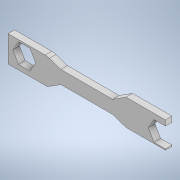
# Autodesk Inventor part: Whack01
Saved by Autodesk Inventor 2020.2 (Build 242310000, 310)
## iProperties
Created: 2019-11-16
Part Number: Whack01
Material: Generic
Document SubType Name: Modeling
Designer: steele
Density: 1 g/cm^3
Appearance: Default
Author: steele
Autodesk Inventor part; units mm, degrees
ref_plane "YZ Plane" through (0, 0, 0) normal (1, 0, 0) x (0, 1, 0)
ref_plane "XZ Plane" through (0, 0, 0) normal (0, 1, 0) x (-1, 0, 0)
ref_plane "XY Plane" through (0, 0, 0) normal (0, 0, 1) x (1, 0, 0)
sketch "Sketch1" plane through (0, 0, 0) normal (0, 0, 1) x (1, 0, 0)
  line L0 (76.176, -10.7873) -> (76.176, 14.6127)
  line L1 (-76.176, 10.7873) -> (-76.176, -14.6127)
  line L2 (-76.176, -14.6127) -> (76.176, 14.6127) construction
  line L3 (76.176, -10.7873) -> (-76.176, 10.7873) construction
  line L4 (76.176, 9.4269) -> (81.6753, -0.0981)
  line L5 (81.6753, -0.0981) -> (76.176, -9.6231)
  line L6 (76.176, -9.6231) -> (65.1775, -9.6231)
  line L7 (65.1775, -9.6231) -> (59.6782, -0.0981)
  line L8 (59.6782, -0.0981) -> (65.1775, 9.4269)
  line L9 (65.1775, 9.4269) -> (76.176, 9.4269)
  line L10 (76.176, 9.4269) -> (76.176, -9.6231) construction
  line L11 (-54.9157, 9.1213) -> (-49.4164, -0.4037)
  line L12 (-49.4164, -0.4037) -> (-54.9157, -9.9287)
  line L13 (-54.9157, -9.9287) -> (-65.9142, -9.9287)
  line L14 (-65.9142, -9.9287) -> (-71.4135, -0.4037)
  line L15 (-71.4135, -0.4037) -> (-65.9142, 9.1213)
  line L16 (-65.9142, 9.1213) -> (-54.9157, 9.1213)
  line L17 (-76.176, -14.6127) -> (-38.076, -14.6127) construction
  line L18 (-38.076, -14.6127) -> (-38.076, 10.7873) construction
  line L19 (-40.1744, 10.7873) -> (-76.176, 10.7873) construction
  line L20 (-76.176, 10.7873) -> (-76.176, -14.6127) construction
  line L21 (76.176, 14.6127) -> (38.076, 14.6127) construction
  line L22 (38.076, 14.6127) -> (38.076, -10.7873) construction
  line L23 (38.076, -10.7873) -> (76.176, -10.7873) construction
  line L24 (76.176, -10.7873) -> (76.176, 14.6127) construction
  line L25 (-25.0148, -6.35) -> (25.0148, -6.35) construction
  line L26 (25.0148, -6.35) -> (25.0148, 6.35) construction
  line L27 (25.0148, 6.35) -> (-25.0148, 6.35) construction
  line L28 (-25.0148, 6.35) -> (-25.0148, -6.35) construction
  line L29 (-25.0148, -6.35) -> (25.0148, 6.35) construction
  line L30 (25.0148, -6.35) -> (-25.0148, 6.35) construction
  line L31 (-36.0891, 10.1123) -> (-25.0148, 6.35)
  line L32 (25.0148, 6.35) -> (38.076, 14.6127)
  line L33 (25.0148, 6.35) -> (-25.0148, 6.35)
  line L34 (-38.076, -14.6127) -> (-25.0148, -6.35)
  line L35 (-25.0148, -6.35) -> (25.0148, -6.35)
  line L36 (25.0148, -6.35) -> (38.076, -10.7873)
  line L37 (76.176, 14.6127) -> (38.076, 14.6127)
  line L38 (-38.076, 10.7873) -> (-76.176, 10.7873)
  line L39 (-76.176, -14.6127) -> (-38.076, -14.6127)
  line L40 (38.076, -10.7873) -> (76.176, -10.7873)
  arc A0 (-36.0891, 10.1123) -> (-40.1744, 10.7873) centre (-40.1744, -1.9127) ccw
  point P0 (0, 0)
  point P1 (70.6767, -0.0981)
  point P2 (-60.415, -0.4037)
  point P3 (76.176, -9.6231)
  point P4 (76.176, 9.4269)
  dimension "totalLength" = 152.4
  dimension "d1" = 25.4
  dimension "d2" = 19.05
  dimension "d3" = 4.7625
  dimension "d4" = 19.05
  dimension "d5" = 38.1
  dimension "d6" = 38.1
  dimension "d8" = 12.7
  dimension "d9" = 12.7
  constraints: 82 end point, 13 parallel, 7 horizontal, 6 perpendicular, 4 midpoint, 2 collinear, 2 point on circle, 2 point on line, 2 tangent, 1 centre point, 26 other
  measures "totalLength" distance of L1.end L0.start
  measures "d1" distance of L0.end L0.start
  measures "d2" distance between parallel lines of L6 L9
  measures "d3" distance from line of L1 L14.end
  measures "d4" distance between parallel lines of L13 L16
  measures "d5" distance of L19.end L18.end
  measures "d6" distance of L23.end L22.end
  measures "d8" distance of L27.end L25.start
  measures "d9" radius of A0
extrude "Extrusion1" add sketch "Sketch1" along normal mid plane 6.35 contours L40 L36 L35 L34 L39 L1 L38 A0 L31 L33 L32 L37 L0 L9 L8 L7 L6
body "Solid1"
